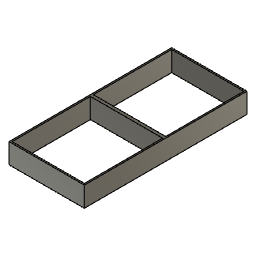
pizarra (Autodesk Fusion 360 archive; units mm, degrees)
design "Grilla F"
Autodesk Fusion 360 part; units mm, degrees
(part 1 of 4)
sketch "Sketch1" plane through (0, 0, 0) normal (0, 0, 1) x (1, 0, 0)
  line L0 (36.035, 39) -> (-36.035, 39)
  line L1 (-36.035, 39) -> (-36.035, -39)
  line L2 (-36.035, -39) -> (36.035, -39)
  line L3 (36.035, -39) -> (36.035, 39)
  line L4 (36.035, 39) -> (-36.035, -39) construction
  line L5 (-36.035, 39) -> (36.035, -39) construction
  line L6 (36.035, -39) -> (-36.035, -39)
  line L7 (-36.035, -42) -> (36.035, -42)
  line L8 (-36.035, -42) -> (36.035, -42)
  line L9 (36.035, -42) -> (36.035, -120)
  line L10 (36.035, -120) -> (-36.035, -120)
  line L11 (-36.035, -120) -> (-36.035, -42)
  line L12 (36.035, -120) -> (-36.035, -120)
  line L13 (-36.035, -121.5) -> (37.465, -121.5)
  line L14 (36.035, 39) -> (-36.035, 39)
  line L15 (-36.035, 40.5) -> (37.465, 40.5)
  line L16 (-36.035, 40.5) -> (-37.535, 40.5)
  line L17 (-37.535, 40.5) -> (-37.535, -121.5)
  line L18 (-37.535, -121.5) -> (-36.035, -121.5)
  line L19 (36.035, -120) -> (36.035, -42)
  line L20 (36.035, -39) -> (36.035, 39)
  line L21 (-36.035, -120) -> (-36.035, -42)
  line L22 (-36.035, -39) -> (-36.035, 39)
  line L23 (-37.535, -126.0665) -> (37.465, -126.0665)
  line L24 (37.465, 40.5) -> (37.465, -121.5)
  line L25 (35.965, -120) -> (35.965, -42)
  line L26 (35.965, -39) -> (35.965, 39)
  dimension "d9" = 72.07
  dimension "d10" = 78
  dimension "d11" = 3
  dimension "d12" = 78
  dimension "d14" = 159
  dimension "d17" = 1.5
  dimension "d20" = 75
  constraint horizontal L0
  constraint perpendicular L0 L1
  constraint parallel L0 L2
  constraint parallel L1 L3
  constraint coincident L4 origin
  constraint coincident L5 origin
  constraint horizontal L6
  constraint horizontal L7
  constraint horizontal L8
  constraint vertical L9
  constraint horizontal L10
  constraint vertical L11
  constraint vertical L19
  constraint horizontal L12
  constraint horizontal L13
  constraint horizontal L14
  constraint horizontal L15
  constraint horizontal L16
  constraint vertical L17
  constraint horizontal L18
  constraint vertical L21
  constraint collinear L19 L20
  constraint collinear L21 L22
  constraint perpendicular L17 L23
  constraint vertical L25
  constraint vertical L24
  constraint coincident L0 L26.end
  constraint coincident L7 L25.end
  constraint coincident L2 L26.start
  constraint collinear L25 L26
  constraint coincident L10 L25.start
  measures "d9" distance of L1.end L2.end
  measures "d10" distance of L0.end L1.end
  measures "d11" distance of L2.end L7.end
  measures "d12" distance of L7.start L10.end
  measures "d14" distance of L0.start L9.end
  measures "d17" distance of L15.start L16.end
  measures "d20" distance of L23.start L23.end
extrude "Extrude2" add sketch "Sketch1" along normal blind 20

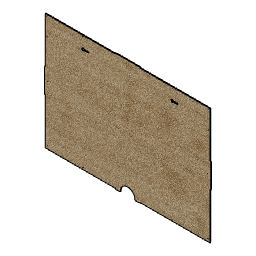
design "F.Panel Trasero.v2"
Autodesk Fusion 360 part; units mm, degrees
ref_plane "WorkPlane1" through (0, 80, 0) normal (0, 1, 0) x (0, 0, 1)
sketch "Sketch1" plane through (0, 80, 0) normal (0, 1, 0) x (1, 0, 0)
  line L0 (337.5, -238.5) -> (-337.5, 238.5) construction
  line L1 (-337.5, -238.5) -> (337.5, 238.5) construction
  line L2 (0, 0) -> (50, 0)
  line L3 (0, 0) -> (-50, 0)
  line L4 (0, 0) -> (0, -50)
  line L5 (0, 0) -> (0, 50)
  line L6 (50, -238.5) -> (50, -241.5)
  line L7 (50, -241.5) -> (-50, -241.5)
  line L8 (-50, -241.5) -> (-50, -238.5)
  line L9 (-337.5, -50) -> (-340.5, -50)
  line L10 (-340.5, -50) -> (-340.5, 50)
  line L11 (-340.5, 50) -> (-337.5, 50)
  line L12 (337.5, -50) -> (340.5, -50)
  line L13 (340.5, -50) -> (340.5, 50)
  line L14 (340.5, 50) -> (337.5, 50)
  line L15 (50, 238.5) -> (50, 241.5)
  line L16 (-50, 241.5) -> (-50, 238.5)
  arc A0 (-29.8496, 241.5) -> (29.8496, 241.5) centre (0, 238.5) ccw
  line L17 (50, 241.5) -> (29.8496, 241.5)
  line L18 (-29.8496, 241.5) -> (-50, 241.5)
  line L19 (-337.5, 238.5) -> (-50, 238.5)
  line L20 (50, 238.5) -> (337.5, 238.5)
  line L21 (337.5, 238.5) -> (337.5, 50)
  line L22 (337.5, -50) -> (337.5, -238.5)
  line L23 (337.5, -238.5) -> (50, -238.5)
  line L24 (-50, -238.5) -> (-337.5, -238.5)
  line L25 (-337.5, -238.5) -> (-337.5, -50)
  line L26 (-337.5, 50) -> (-337.5, 238.5)
  dimension "d14" = 675
  dimension "d15" = 477
  dimension "d16" = 50
  dimension "d17" = 50
  dimension "d18" = 50
  dimension "d19" = 50
  dimension "d20" = 3
  dimension "d21" = 3
  dimension "d22" = 100
  dimension "d23" = 3
  dimension "d24" = 3
  dimension "d25" = 60
  constraint horizontal L23
  constraint perpendicular L23 L25
  constraint parallel L19 L23
  constraint parallel L21 L25
  constraint coincident L0 L2.start
  constraint coincident L1 L2.start
  constraint coincident L2.start L3.start
  constraint horizontal L2
  constraint parallel L2 L3
  constraint perpendicular L3 L4
  constraint perpendicular L3 L5
  constraint vertical L6
  constraint horizontal L7
  constraint vertical L8
  constraint coincident L8.end L23
  constraint horizontal L9
  constraint vertical L10
  constraint horizontal L11
  constraint horizontal L12
  constraint vertical L13
  constraint horizontal L14
  constraint coincident L12.start L21
  constraint vertical L15
  constraint horizontal L17
  constraint vertical L16
  constraint coincident A0.start L17
  constraint collinear L17 L18
  constraint collinear L19 L20
  constraint collinear L21 L22
  constraint collinear L23 L24
  constraint collinear L25 L26
  measures "d14" distance of L0.end L1.end
  measures "d15" distance of L1.start L0.end
  measures "d16" distance of L2.start L2.end
  measures "d17" distance of L2.start L3.end
  measures "d18" distance of L2.start L4.end
  measures "d19" distance of L2.start L5.end
  measures "d20" distance of L8.end L7.end
  measures "d21" distance of L9.start L9.end
  measures "d22" distance of L9.start L11.end
  measures "d23" distance of L12.start L12.end
  measures "d24" distance of L16.end L16.start
  measures "d25" diameter of A0
extrude "Extrude3" add sketch "Sketch1" along normal blind 3
ref_plane "WorkPlane2" through (0, 80, 0) normal (0, -1, 0) x (-1, 0, 0)
sketch "Sketch2" plane through (0, 80, 0) normal (0, -1, 0) x (1, 0, 0)
  line L0 (340.5, 50) -> (337.5, 50)
  line L1 (337.5, 50) -> (337.5, 238.5)
  line L2 (337.5, 238.5) -> (50, 238.5)
  line L3 (50, 238.5) -> (50, 241.5)
  line L4 (50, 241.5) -> (-50, 241.5)
  line L5 (-50, 241.5) -> (-50, 238.5)
  line L6 (-50, 238.5) -> (-337.5, 238.5)
  line L7 (-337.5, 238.5) -> (-337.5, 50)
  line L8 (-337.5, 50) -> (-340.5, 50)
  line L9 (-340.5, 50) -> (-340.5, -50)
  line L10 (-340.5, -50) -> (-337.5, -50)
  line L11 (-337.5, -50) -> (-337.5, -238.5)
  line L12 (-337.5, -238.5) -> (-50, -238.5)
  line L13 (-50, -238.5) -> (-50, -241.5)
  line L14 (-50, -241.5) -> (-29.8496, -241.5)
  arc A0 (29.8496, -241.5) -> (-29.8496, -241.5) centre (0, -238.5) ccw
  line L15 (29.8496, -241.5) -> (50, -241.5)
  line L16 (50, -241.5) -> (50, -238.5)
  line L17 (50, -238.5) -> (337.5, -238.5)
  line L18 (337.5, -238.5) -> (337.5, -50)
  line L19 (337.5, -50) -> (340.5, -50)
  line L20 (340.5, -50) -> (340.5, 50)
ref_plane "WorkPlane3" through (0, 80, 0) normal (0, -1, 0) x (-1, 0, 0)
sketch "Sketch3" plane through (0, 80, 0) normal (0, -1, 0) x (1, 0, 0)
  circle A0 centre (-182.9674, -231.5) radius 1
  circle A1 centre (183.0674, -231.5) radius 1
  circle A2 centre (-328.5, -226.5) radius 1
  line L0 (473.5457, 191.5) -> (473.5457, 128.3996) construction
  circle A3 centre (326.5, 2.556) radius 1
  circle A4 centre (328.5, -226.5) radius 1
  line L1 (-50, 238.5) -> (-50, 241.5)
  line L2 (-340.5, -50) -> (-337.5, -50)
  line L3 (-330.5, 141.5) -> (-330.5, 159.5)
  line L4 (-330.5, 159.5) -> (-340.5, 159.5)
  line L5 (-340.5, 141.5) -> (-330.5, 141.5)
  circle A5 centre (-330.5, 232.5) radius 1
  line L6 (-330.5, 232.5) -> (-340.5, 232.5)
  line L7 (-50, 241.5) -> (-50, 238.5)
  circle A6 centre (183.022, 233.5) radius 1
  circle A7 centre (330.5, 159.5) radius 1
  circle A8 centre (330.5, 232.5) radius 1
  line L8 (330.5, 159.5) -> (338.4264, 160.0934)
  circle A9 centre (-183.0217, 233.5) radius 1
  line L9 (-330.5, 241.5) -> (-330.5, 232.5)
  line L10 (-340.5, 159.5) -> (-340.5, 141.5)
  line L11 (340.5, -50) -> (337.5, -50)
  line L12 (-337.5, -50) -> (-340.5, -50)
  line L13 (337.5, -50) -> (340.5, -50)
  line L14 (-340.5, 232.5) -> (-340.5, 241.5)
  line L15 (-340.5, 241.5) -> (-330.5, 241.5)
  circle A10 centre (-330.5, 159.3463) radius 1
  line L16 (-161.02, 186.5) -> (-178.0217, 186.5)
  line L17 (-178.0217, 190.5) -> (-161.02, 190.5)
  arc A11 (-161.02, 186.5) -> (-161.02, 190.5) centre (-161.02, 188.5) ccw
  arc A12 (-178.5672, 190.7709) -> (-178.5672, 186.2291) centre (-183.0217, 188.5) ccw
  arc A13 (205.0238, 186.5) -> (205.0238, 190.5) centre (205.0238, 188.5) ccw
  line L18 (188.022, 190.5) -> (205.0238, 190.5)
  line L19 (205.0238, 186.5) -> (188.022, 186.5)
  arc A14 (187.4765, 190.7709) -> (187.4765, 186.2291) centre (183.022, 188.5) ccw
  arc A15 (187.942, 186.5016) -> (187.4765, 186.2291) centre (187.922, 186.002) ccw
  arc A16 (187.942, 186.5016) -> (188.022, 186.5) centre (188.022, 188.5) ccw
  arc A17 (187.4765, 190.7709) -> (187.942, 190.4984) centre (187.922, 190.998) ccw
  arc A18 (188.022, 190.5) -> (187.942, 190.4984) centre (188.022, 188.5) ccw
  line L20 (-178.5672, 190.7709) -> (-178.0217, 190.5)
  line L21 (-178.5672, 186.2291) -> (-178.0217, 186.5)
  line L22 (340.5, 50) -> (337.5, 50)
  line L23 (337.5, 50) -> (337.5, 238.5)
  line L24 (337.5, 238.5) -> (50, 238.5)
  line L25 (50, 238.5) -> (50, 241.5)
  line L26 (50, 241.5) -> (-50, 241.5)
  line L27 (-50, 241.5) -> (-50, 238.5)
  line L28 (-50, 238.5) -> (-337.5, 238.5)
  line L29 (-337.5, 238.5) -> (-337.5, 50)
  line L30 (-337.5, 50) -> (-340.5, 50)
  line L31 (-340.5, 50) -> (-340.5, -50)
  line L32 (-340.5, -50) -> (-337.5, -50)
  line L33 (-337.5, -50) -> (-337.5, -238.5)
  line L34 (-337.5, -238.5) -> (-50, -238.5)
  line L35 (-50, -238.5) -> (-50, -241.5)
  line L36 (-50, -241.5) -> (-29.8496, -241.5)
  arc A19 (29.8496, -241.5) -> (-29.8496, -241.5) centre (0, -238.5) ccw
  line L37 (29.8496, -241.5) -> (50, -241.5)
  line L38 (50, -241.5) -> (50, -238.5)
  line L39 (50, -238.5) -> (337.5, -238.5)
  line L40 (337.5, -238.5) -> (337.5, -50)
  line L41 (337.5, -50) -> (340.5, -50)
  line L42 (340.5, -50) -> (340.5, 50)
  line L43 (-340.5, 241.5) -> (340.5, 241.5)
  line L44 (340.5, 241.5) -> (340.5, 141.5)
  line L45 (340.5, 141.5) -> (-340.5, 141.5)
  line L46 (-340.5, 141.5) -> (-340.5, 241.5)
  line L47 (-183.0217, 188.5) -> (-183.0217, 241.5)
  line L48 (183.022, 188.5) -> (183.022, 241.5)
  line L49 (-340.5, 3.0863) -> (-326.5, 3.0863)
  circle A20 centre (-326.5, 3.0863) radius 1
  line L50 (-337.5, -238.5) -> (-337.5, -241.5)
  line L51 (-337.5, -238.5) -> (-340.5, -238.5)
  line L52 (-337.5, -241.5) -> (-316, -241.5)
  line L53 (-340.5, -238.5) -> (-340.5, -223)
  point P0 (-3, -3)
  point P1 (-3, -3)
  point P2 (-3, -3)
  dimension "d49" = 2
  dimension "d50" = 2
  dimension "d67" = 2
  dimension "d109" = 2
  dimension "d112" = 2
  dimension "d6" = 10
  dimension "d7" = 9
  dimension "d8" = 10
  dimension "d9" = 18
  dimension "d137" = 2
  dimension "d138" = 2
  dimension "d139" = 2
  dimension "d140" = 2
  dimension "d141" = 2
  dimension "d142" = 2
  dimension "d143" = 5
  dimension "d144" = 5
  dimension "d152" = 681
  dimension "d153" = 100
  dimension "d154" = 10
  dimension "d155" = 9
  dimension "d156" = 8
  dimension "d157" = 10
  dimension "d158" = 18
  dimension "d159" = 53
  dimension "d160" = 157.4783
  dimension "d161" = 8
  dimension "d162" = 157.478
  dimension "d163" = 53
  dimension "d165" = 14
  dimension "d166" = 9
  dimension "d167" = 12
  dimension "d168" = 7
  dimension "d169" = 7
  dimension "d170" = 9
  dimension "d171" = 12
  dimension "d172" = 14
  dimension "d173" = 2
  dimension "d179" = 3
  dimension "d180" = 3
  constraint horizontal L43
  constraint vertical L44
  constraint horizontal L45
  constraint vertical L46
  constraint coincident A12.centre L47.start
  constraint coincident L43 L47.end
  constraint perpendicular L43 L47
  constraint coincident A14.centre L48.start
  constraint coincident L43 L48.end
  constraint perpendicular L43 L48
  constraint coincident L31 L49.start
  constraint perpendicular L31 L49
  constraint coincident L49.end A20.centre
  constraint coincident L33.end L34.start
  constraint perpendicular L34 L50
  constraint perpendicular L33 L51
  constraint perpendicular L50 L52
  constraint perpendicular L51 L53
  measures "d49" diameter of A0
  measures "d50" diameter of A1
  measures "d67" diameter of A2
  measures "d109" diameter of A3
  measures "d112" diameter of A4
  measures "d6" distance of L14.end L9.start
  measures "d7" distance of L6.end L14.end
  measures "d8" distance of L3.start L5.start
  measures "d9" distance of L4.end L5.start
  measures "d137" diameter of A6
  measures "d138" diameter of A9
  measures "d139" diameter of A5
  measures "d140" diameter of A10
  measures "d141" diameter of A8
  measures "d142" diameter of A7
  measures "d143" radius of A12
  measures "d144" radius of A14
  measures "d152" distance of L14.end L43.end
  measures "d153" distance of L14.end L5.start
  measures "d154" distance of A8.centre L44
  measures "d155" distance of A8.centre L43
  measures "d156" distance of A6.centre L43
  measures "d157" distance of A7.centre L44
  measures "d158" distance of A7.centre L45
  measures "d159" distance of A12.centre L43
  measures "d160" distance of A12.centre L46
  measures "d161" distance of A9.centre L43
  measures "d162" distance of A14.centre L44
  measures "d163" distance of A14.centre L43
  measures "d165" distance of A3.centre L42
  measures "d166" distance of A2.centre L33
  measures "d167" distance of A2.centre L34
  measures "d168" distance of A0.centre L34
  measures "d169" distance of A1.centre L39
  measures "d170" distance of A4.centre L40
  measures "d171" distance of A4.centre L39
  measures "d172" distance of L49.start L49.end
  measures "d173" diameter of A20
  measures "d179" distance of L33.end L50.end
  measures "d180" distance of L33.end L51.end
extrude "Extrude4" cut sketch "Sketch3" against normal blind 50 contours A0 | A1 | A2 | A3 | A4 | A5 L6 L9 | A5 L6 L9 | L3 L4 A10 | L3 L4 A10 | A6 L48 | A6 L48 | A7 | A8 | A9 L47 | A9 L47 | L16 L17 A11 A12 L20 L21 | A13 L18 L19 A14 A15 A16 A17 A18 | A20
ref_plane "WorkPlane4" through (0, 80, 0) normal (0, -1, 0) x (-1, 0, 0)
sketch "Sketch5" plane through (0, 80, 0) normal (0, -1, 0) x (1, 0, 0)
  circle A0 centre (330.5, 232.5) radius 1
  circle A1 centre (-330.5, 232.5) radius 1
  circle A2 centre (-328.5, -226.5) radius 1
  circle A3 centre (-182.9674, -231.5) radius 1
  circle A4 centre (-330.5, 159.3463) radius 1
  circle A5 centre (330.5, 159.5) radius 1
  line L0 (-178.0217, 186.5) -> (-178.5672, 186.2291)
  arc A6 (-178.5672, 190.7709) -> (-178.5672, 186.2291) centre (-183.0217, 188.5) ccw
  line L1 (-178.5672, 190.7709) -> (-178.0217, 190.5)
  line L2 (-178.0217, 190.5) -> (-161.02, 190.5)
  arc A7 (-161.02, 186.5) -> (-161.02, 190.5) centre (-161.02, 188.5) ccw
  line L3 (-161.02, 186.5) -> (-178.0217, 186.5)
  circle A8 centre (-183.0217, 233.5) radius 1
  circle A9 centre (326.5, 2.556) radius 1
  circle A10 centre (183.0674, -231.5) radius 1
  circle A11 centre (328.5, -226.5) radius 1
  circle A12 centre (183.022, 233.5) radius 1
  line L4 (188.022, 190.5) -> (205.0238, 190.5)
  arc A13 (205.0238, 186.5) -> (205.0238, 190.5) centre (205.0238, 188.5) ccw
  line L5 (205.0238, 186.5) -> (188.022, 186.5)
  arc A14 (187.942, 186.5016) -> (188.022, 186.5) centre (188.022, 188.5) ccw
  arc A15 (187.942, 186.5016) -> (187.4765, 186.2291) centre (187.922, 186.002) ccw
  arc A16 (187.4765, 190.7709) -> (187.4765, 186.2291) centre (183.022, 188.5) ccw
  arc A17 (187.4765, 190.7709) -> (187.942, 190.4984) centre (187.922, 190.998) ccw
  arc A18 (188.022, 190.5) -> (187.942, 190.4984) centre (188.022, 188.5) ccw
  line L6 (340.5, 50) -> (337.5, 50)
  line L7 (337.5, 50) -> (337.5, 238.5)
  line L8 (337.5, 238.5) -> (50, 238.5)
  line L9 (50, 238.5) -> (50, 241.5)
  line L10 (50, 241.5) -> (-50, 241.5)
  line L11 (-50, 241.5) -> (-50, 238.5)
  line L12 (-50, 238.5) -> (-337.5, 238.5)
  line L13 (-337.5, 238.5) -> (-337.5, 50)
  line L14 (-337.5, 50) -> (-340.5, 50)
  line L15 (-340.5, 50) -> (-340.5, -50)
  line L16 (-340.5, -50) -> (-337.5, -50)
  line L17 (-337.5, -50) -> (-337.5, -238.5)
  line L18 (-337.5, -238.5) -> (-50, -238.5)
  line L19 (-50, -238.5) -> (-50, -241.5)
  line L20 (-50, -241.5) -> (-29.8496, -241.5)
  arc A19 (29.8496, -241.5) -> (-29.8496, -241.5) centre (0, -238.5) ccw
  line L21 (29.8496, -241.5) -> (50, -241.5)
  line L22 (50, -241.5) -> (50, -238.5)
  line L23 (50, -238.5) -> (337.5, -238.5)
  line L24 (337.5, -238.5) -> (337.5, -50)
  line L25 (337.5, -50) -> (340.5, -50)
  line L26 (340.5, -50) -> (340.5, 50)
  line L27 (-337.5, 238.5) -> (-337.5, 241.5)
  line L28 (-337.5, 238.5) -> (-340.5, 238.5)
  line L29 (337.5, 238.5) -> (340.5, 238.5)
  line L30 (-340.5, 241.5) -> (340.5, 241.5)
  line L31 (340.5, 241.5) -> (340.5, 141.5)
  line L32 (340.5, 141.5) -> (-340.5, 141.5)
  line L33 (-340.5, 141.5) -> (-340.5, 241.5)
  circle A20 centre (-326.5, 3.0863) radius 1
  dimension "d174" = 3
  dimension "d175" = 3
  dimension "d176" = 3
  dimension "d177" = 100
  dimension "d178" = 681
  constraint coincident L12.end L13.start
  constraint perpendicular L12 L27
  constraint perpendicular L13 L28
  constraint coincident L7.end L8.start
  constraint perpendicular L7 L29
  constraint horizontal L30
  constraint vertical L31
  constraint horizontal L32
  constraint vertical L33
  measures "d174" distance of L12.end L27.end
  measures "d175" distance of L12.end L28.end
  measures "d176" distance of L7.end L29.end
  measures "d177" distance of L30.start L32.end
  measures "d178" distance of L30.start L30.end

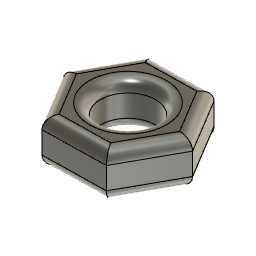
design "N.Perno Alen.v2"
Autodesk Fusion 360 part; units mm, degrees
sketch "Sketch1" plane through (0, 0, 0) normal (0, 0, 1) x (1, 0, 0)
  line L0 (-1.4906, 2.4721) -> (-2.8862, -0.0549)
  line L1 (-2.8862, -0.0549) -> (-1.3956, -2.527)
  line L2 (-1.3956, -2.527) -> (1.4906, -2.4721)
  line L3 (1.4906, -2.4721) -> (2.8862, 0.0549)
  line L4 (2.8862, 0.0549) -> (1.3956, 2.527)
  line L5 (1.3956, 2.527) -> (-1.4906, 2.4721)
  circle A0 centre (0, 0) radius 1.25
  dimension "d1" = 2.5
  dimension "d2" = 2.5
  constraint coincident A0.centre origin
  measures "d1" distance of A0.centre L5
  measures "d2" diameter of A0
extrude "Extrude1" add sketch "Sketch1" along normal blind 2
fillet "Fillet1" radius 0.5 1 faces at (0.0628, -2.0819, 2)
fillet "Fillet2" radius 0.5 1 faces at (0.0628, -2.0819, 0)

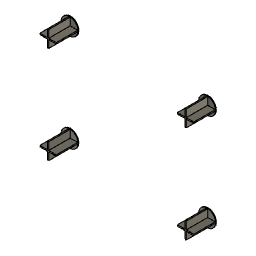
design "Cruceta para fondo.v3"
Autodesk Fusion 360 part; units mm, degrees
sketch "Sketch1" plane through (0, 0, 0) normal (0, 1, 0) x (1, 0, 0)
  line L0 (337.5, -238.5) -> (-337.5, -238.5)
  line L1 (-337.5, -238.5) -> (-337.5, 238.5)
  line L2 (-337.5, 238.5) -> (337.5, 238.5)
  line L3 (337.5, 238.5) -> (337.5, -238.5)
  line L4 (0, 0) -> (-163.3332, -115.4221) construction
  circle A0 centre (-163.3332, -115.4221) radius 20
  circle A1 centre (163.3332, -115.4221) radius 20
  circle A2 centre (-163.3332, 115.4221) radius 20
  circle A3 centre (163.3332, 115.4221) radius 20
  line L5 (-161.8332, -134.9221) -> (-164.8332, -134.9221)
  line L6 (-164.8332, -95.9221) -> (-161.8332, -95.9221)
  line L7 (-161.8332, -134.9221) -> (-164.8332, -95.9221) construction
  line L8 (-164.8332, -134.9221) -> (-161.8332, -95.9221) construction
  line L9 (-182.8332, -116.9221) -> (-182.8332, -113.9221)
  line L10 (-143.8332, -113.9221) -> (-143.8332, -116.9221)
  line L11 (-143.8332, -116.9221) -> (-182.8332, -113.9221) construction
  line L12 (-182.8332, -116.9221) -> (-143.8332, -113.9221) construction
  line L13 (-337.5, -238.5) -> (-164.8332, -116.4821) construction
  line L14 (-163.3332, -115.4221) -> (337.5, 238.5) construction
  line L15 (-164.8332, -134.9221) -> (-164.8332, -116.9221) construction
  line L16 (-143.8332, -116.9221) -> (-161.8332, -116.9221) construction
  line L17 (-164.8332, -116.9221) -> (-182.8332, -116.9221) construction
  line L18 (-161.8332, -116.9221) -> (-161.8332, -134.9221) construction
  line L19 (-161.8332, -95.9221) -> (-161.8332, -113.9221) construction
  line L20 (-182.8332, -113.9221) -> (-164.8332, -113.9221) construction
  line L21 (-161.8332, -113.9221) -> (-143.8332, -113.9221) construction
  line L22 (-164.8332, -113.9221) -> (-164.8332, -95.9221) construction
  point P0 (-163.3332, -115.4221)
  point P1 (-163.3332, -115.4221)
  dimension "d1" = 675
  dimension "d2" = 477
  dimension "d3" = 200
  dimension "d4" = 200
  dimension "d5" = 200
  dimension "d6" = 200
  dimension "d7" = 40
  dimension "d8" = 40
  dimension "d9" = 40
  dimension "d10" = 40
  dimension "d11" = 3
  dimension "d12" = 39
  dimension "d13" = 3
  dimension "d14" = 39
  constraint horizontal L0
  constraint perpendicular L0 L1
  constraint parallel L0 L2
  constraint parallel L1 L3
  constraint coincident L4.start L13
  constraint coincident L4.start origin
  constraint coincident P1 L13
  constraint coincident P1 P0
  constraint horizontal L5
  constraint perpendicular L5 L15
  constraint parallel L5 L6
  constraint parallel L15 L19
  constraint coincident L7 P1
  constraint coincident L8 P1
  constraint horizontal L16
  constraint perpendicular L9 L16
  constraint parallel L16 L20
  constraint parallel L9 L10
  constraint coincident L11 P1
  constraint coincident L12 P1
  constraint collinear L13 L14
  constraint coincident L15.end L16
  constraint collinear L16 L17
  constraint coincident L16.end L19
  constraint collinear L18 L19
  constraint coincident L19.end L20
  constraint collinear L20 L21
  measures "d1" distance of L1.end L2.end
  measures "d2" distance of L0.end L1.end
  measures "d3" distance of L4.start P1
  measures "d4" distance of L4.start A1.centre
  measures "d5" distance of L4.start A2.centre
  measures "d6" distance of L4.start A3.centre
  measures "d7" diameter of A0
  measures "d8" diameter of A1
  measures "d9" diameter of A2
  measures "d10" diameter of A3
  measures "d11" distance of L6.start L6.end
  measures "d12" distance of L9.end L10.start
  measures "d13" distance of L9.start L9.end
  measures "d14" distance of L5.start L6.end
extrude "Extrude1" add sketch "Sketch1" along normal blind 2 contours A0 | A1 | A2 | A3 makes body 1 at (-164.4526, 0, -120.9941) makes body 2 at (160.7303, 0, 116.3496) makes body 3 at (-163.5939, 0, 118.7453) makes body 4 at (162.2137, 0, -120.9941)
ref_plane "WorkPlane1" through (-163.3332, 0, 115.4221) normal (0, -1, 0) x (-1, 0, 0)
sketch "Sketch2" plane through (-163.3332, 0, 115.4221) normal (0, -1, 0) x (1, 0, 0)
  line L0 (1.5, 19.5) -> (-1.5, 19.5)
  line L1 (-1.5, 19.5) -> (-1.5, 1.5)
  line L2 (1.5, 1.5) -> (1.5, 19.5)
  line L3 (-1.5, 1.5) -> (-19.5, 1.5)
  line L4 (-19.5, 1.5) -> (-19.5, -1.5)
  line L5 (-19.5, -1.5) -> (-1.5, -1.5)
  line L6 (19.5, 1.5) -> (1.5, 1.5)
  line L7 (19.5, -1.5) -> (19.5, 1.5)
  line L8 (1.5, -1.5) -> (19.5, -1.5)
  line L9 (1.5, -19.5) -> (1.5, -1.5)
  line L10 (-1.5, -19.5) -> (1.5, -19.5)
  line L11 (-1.5, -1.5) -> (-1.5, -19.5)
  line L12 (1.5, -1.5) -> (19.5, -1.5)
  line L13 (-1.5, 1.5) -> (-19.5, 1.5)
  line L14 (1.5, 19.5) -> (-1.5, 19.5)
  line L15 (-19.5, -1.5) -> (-1.5, -1.5)
  line L16 (-1.5, -1.5) -> (-1.5, -19.5)
  line L17 (19.5, 1.5) -> (1.5, 1.5)
  line L18 (1.5, 1.5) -> (1.5, 19.5)
  line L19 (19.5, -1.5) -> (19.5, 1.5)
  line L20 (-1.5, -19.5) -> (1.5, -19.5)
  line L21 (-1.5, 19.5) -> (-1.5, 1.5)
  line L22 (1.5, -19.5) -> (1.5, -1.5)
  line L23 (-19.5, 1.5) -> (-19.5, -1.5)
  circle A0 centre (0, 0) radius 20
  circle A1 centre (326.6664, 0) radius 20
  circle A2 centre (326.6664, -230.8443) radius 20
  circle A3 centre (0, -230.8443) radius 20
  line L24 (325.1664, -19.5) -> (328.1664, -19.5)
  line L25 (325.1664, 19.5) -> (325.1664, 1.5)
  line L26 (307.1664, -1.5) -> (325.1664, -1.5)
  line L27 (307.1664, -1.5) -> (325.1664, -1.5)
  line L28 (325.1664, -1.5) -> (325.1664, -19.5)
  line L29 (346.1664, -1.5) -> (346.1664, 1.5)
  line L30 (328.1664, -19.5) -> (328.1664, -1.5)
  line L31 (307.1664, 1.5) -> (307.1664, -1.5)
  line L32 (346.1664, 1.5) -> (328.1664, 1.5)
  line L33 (328.1664, 19.5) -> (325.1664, 19.5)
  line L34 (346.1664, -1.5) -> (346.1664, 1.5)
  line L35 (328.1664, 1.5) -> (328.1664, 19.5)
  circle A4 centre (326.6664, 0) radius 20
  line L36 (346.1664, 1.5) -> (328.1664, 1.5)
  line L37 (325.1664, 1.5) -> (307.1664, 1.5)
  line L38 (325.1664, -19.5) -> (328.1664, -19.5)
  line L39 (325.1664, 19.5) -> (325.1664, 1.5)
  line L40 (328.1664, -1.5) -> (346.1664, -1.5)
  line L41 (328.1664, -19.5) -> (328.1664, -1.5)
  line L42 (328.1664, 19.5) -> (325.1664, 19.5)
  line L43 (328.1664, 1.5) -> (328.1664, 19.5)
  line L44 (325.1664, 1.5) -> (307.1664, 1.5)
  line L45 (328.1664, -1.5) -> (346.1664, -1.5)
  line L46 (307.1664, 1.5) -> (307.1664, -1.5)
  line L47 (325.1664, -1.5) -> (325.1664, -19.5)
  line L48 (328.1664, -211.3443) -> (325.1664, -211.3443)
  line L49 (346.1664, -232.3443) -> (346.1664, -229.3443)
  line L50 (328.1664, -229.3443) -> (328.1664, -211.3443)
  line L51 (325.1664, -232.3443) -> (325.1664, -250.3443)
  line L52 (307.1664, -232.3443) -> (325.1664, -232.3443)
  circle A5 centre (326.6664, -230.8443) radius 20
  line L53 (328.1664, -211.3443) -> (325.1664, -211.3443)
  line L54 (307.1664, -229.3443) -> (307.1664, -232.3443)
  line L55 (307.1664, -229.3443) -> (307.1664, -232.3443)
  line L56 (325.1664, -250.3443) -> (328.1664, -250.3443)
  line L57 (328.1664, -250.3443) -> (328.1664, -232.3443)
  line L58 (307.1664, -232.3443) -> (325.1664, -232.3443)
  line L59 (346.1664, -229.3443) -> (328.1664, -229.3443)
  line L60 (328.1664, -229.3443) -> (328.1664, -211.3443)
  line L61 (328.1664, -232.3443) -> (346.1664, -232.3443)
  line L62 (325.1664, -232.3443) -> (325.1664, -250.3443)
  line L63 (328.1664, -250.3443) -> (328.1664, -232.3443)
  line L64 (325.1664, -211.3443) -> (325.1664, -229.3443)
  line L65 (325.1664, -229.3443) -> (307.1664, -229.3443)
  line L66 (325.1664, -211.3443) -> (325.1664, -229.3443)
  line L67 (325.1664, -229.3443) -> (307.1664, -229.3443)
  line L68 (346.1664, -229.3443) -> (328.1664, -229.3443)
  circle A6 centre (326.6664, -230.8443) radius 20
  line L69 (325.1664, -250.3443) -> (328.1664, -250.3443)
  line L70 (346.1664, -232.3443) -> (346.1664, -229.3443)
  line L71 (328.1664, -232.3443) -> (346.1664, -232.3443)
  line L72 (1.5, -211.3443) -> (-1.5, -211.3443)
  line L73 (19.5, -232.3443) -> (19.5, -229.3443)
  line L74 (1.5, -229.3443) -> (1.5, -211.3443)
  line L75 (-1.5, -232.3443) -> (-1.5, -250.3443)
  line L76 (-19.5, -232.3443) -> (-1.5, -232.3443)
  circle A7 centre (0, -230.8443) radius 20
  line L77 (1.5, -211.3443) -> (-1.5, -211.3443)
  line L78 (-19.5, -229.3443) -> (-19.5, -232.3443)
  line L79 (-19.5, -229.3443) -> (-19.5, -232.3443)
  line L80 (-1.5, -250.3443) -> (1.5, -250.3443)
  line L81 (1.5, -250.3443) -> (1.5, -232.3443)
  line L82 (-19.5, -232.3443) -> (-1.5, -232.3443)
  line L83 (19.5, -229.3443) -> (1.5, -229.3443)
  line L84 (1.5, -229.3443) -> (1.5, -211.3443)
  line L85 (1.5, -232.3443) -> (19.5, -232.3443)
  line L86 (-1.5, -232.3443) -> (-1.5, -250.3443)
  line L87 (1.5, -250.3443) -> (1.5, -232.3443)
  line L88 (-1.5, -211.3443) -> (-1.5, -229.3443)
  line L89 (-1.5, -229.3443) -> (-19.5, -229.3443)
  line L90 (-1.5, -211.3443) -> (-1.5, -229.3443)
  line L91 (-1.5, -229.3443) -> (-19.5, -229.3443)
  line L92 (19.5, -229.3443) -> (1.5, -229.3443)
  circle A8 centre (0, -230.8443) radius 20
  line L93 (-1.5, -250.3443) -> (1.5, -250.3443)
  line L94 (19.5, -232.3443) -> (19.5, -229.3443)
  line L95 (1.5, -232.3443) -> (19.5, -232.3443)
  point P0 (306.6664, -230.8443)
  point P1 (326.6664, 0)
  point P2 (326.6664, 0)
  point P3 (326.6664, -230.8443)
  point P4 (326.6664, -230.8443)
  point P5 (0, -230.8443)
  point P6 (0, -230.8443)
extrude "Extrude2" add sketch "Sketch2" along normal blind 51 contours L0 L1 L2 L3 L4 L5 L6 L7 L8 L9 L10 L11 L12 L13 L14 L15 L16 L17 L18 L19 L20 L21 L22 L23 | L24 L25 L26 L27 L28 L29 L30 L31 L32 L33 L34 L35 L36 L37 L38 L39 L40 L41 L42 L43 L44 L45 L46 L47 | L48 L49 L50 L51 L52 L53 L54 L55 L56 L57 L58 L59 L60 L61 L62 L63 L64 L65 L66 L67 L68 L69 L70 L71 bodies 2 3 4
extrude "Extrude3" add sketch "Sketch2" along normal blind 51 contours L72 L73 L74 L75 L76 L77 L78 L79 L80 L81 L82 L83 L84 L85 L86 L87 L88 L89 L90 L91 L92 L93 L94 L95 bodies 1

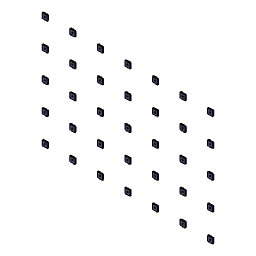
design "onjunto piezas perno"
Autodesk Fusion 360 part; units mm, degrees
sketch "Sketch1" plane through (0, 0, 0) normal (0, 1, 0) x (1, 0, 0)
  circle A0 centre (252, -728) radius 1.75
  circle A1 centre (252, -647) radius 1.75
  line L0 (325.5, -735.5) -> (340.5, -735.5)
  circle A2 centre (252, -566) radius 1.75
  line L1 (259.5, -654.5) -> (259.5, -639.5)
  line L2 (340.5, -636.5) -> (340.5, -639.5)
  line L3 (340.5, -639.5) -> (325.5, -639.5)
  line L4 (340.5, -720.5) -> (325.5, -720.5)
  line L5 (97.5, -735.5) -> (97.5, -720.5)
  circle A3 centre (252, -809) radius 1.75
  line L6 (-340.5, -636.5) -> (340.5, -636.5) construction
  line L7 (178.5, -735.5) -> (178.5, -720.5)
  line L8 (-340.5, -882.5) -> (340.5, -882.5) construction
  line L9 (325.5, -816.5) -> (340.5, -816.5)
  line L10 (-340.5, -960.5) -> (340.5, -960.5) construction
  line L11 (-340.5, -801.5) -> (340.5, -801.5) construction
  line L12 (262.5, -963.5) -> (262.5, -1041.5) construction
  line L13 (340.5, -801.5) -> (340.5, -879.5)
  circle A4 centre (171, -566) radius 1.75
  line L14 (325.5, -801.5) -> (325.5, -816.5)
  line L15 (244.5, -816.5) -> (259.5, -816.5)
  line L16 (340.5, -816.5) -> (340.5, -801.5)
  line L17 (340.5, -717.5) -> (-340.5, -717.5) construction
  line L18 (-340.5, -639.5) -> (340.5, -639.5) construction
  line L19 (19.5, -1041.5) -> (97.5, -1041.5) construction
  line L20 (340.5, -882.5) -> (-340.5, -882.5) construction
  line L21 (-340.5, -558.5) -> (340.5, -558.5) construction
  circle A5 centre (252, -890) radius 1.75
  line L22 (259.5, -897.5) -> (259.5, -882.5)
  line L23 (340.5, -1041.5) -> (-340.5, -1041.5) construction
  line L24 (-340.5, -798.5) -> (340.5, -798.5) construction
  line L25 (100.5, -558.5) -> (97.5, -558.5)
  line L26 (340.5, -798.5) -> (-340.5, -798.5) construction
  line L27 (-340.5, -720.5) -> (340.5, -720.5) construction
  line L28 (16.5, -720.5) -> (1.5, -720.5)
  line L29 (-226.5, -1041.5) -> (-223.5, -1041.5) construction
  line L30 (82.5, -816.5) -> (97.5, -816.5)
  circle A6 centre (171, -890) radius 1.75
  line L31 (-340.5, -639.5) -> (-340.5, -636.5)
  line L32 (97.5, -1041.5) -> (100.5, -1041.5) construction
  line L33 (-340.5, -882.5) -> (-340.5, -879.5)
  circle A7 centre (-153, -809) radius 1.75
  circle A8 centre (-72, -728) radius 1.75
  line L34 (16.5, -816.5) -> (16.5, -801.5)
  line L35 (-64.5, -1041.5) -> (-64.5, -963.5) construction
  line L36 (-160.5, -720.5) -> (-160.5, -735.5)
  line L37 (-160.5, -816.5) -> (-145.5, -816.5)
  circle A9 centre (-72, -890) radius 1.75
  line L38 (1.5, -882.5) -> (1.5, -897.5)
  line L39 (-223.5, -1041.5) -> (-145.5, -1041.5) construction
  line L40 (-145.5, -897.5) -> (-145.5, -882.5)
  line L41 (178.5, -1041.5) -> (181.5, -1041.5) construction
  line L42 (-64.5, -558.5) -> (-79.5, -558.5)
  line L43 (178.5, -1041.5) -> (178.5, -963.5) construction
  line L44 (-145.5, -573.5) -> (-145.5, -558.5)
  line L45 (-145.5, -963.5) -> (-223.5, -963.5)
  circle A10 centre (-153, -566) radius 1.75
  line L46 (178.5, -816.5) -> (178.5, -801.5)
  line L47 (-64.5, -573.5) -> (-64.5, -558.5)
  line L48 (-160.5, -801.5) -> (-160.5, -816.5)
  line L49 (-340.5, -1041.5) -> (-226.5, -1041.5) construction
  line L50 (-145.5, -558.5) -> (-160.5, -558.5)
  line L51 (-160.5, -558.5) -> (-160.5, -573.5)
  line L52 (-61.5, -963.5) -> (-61.5, -1041.5) construction
  line L53 (-142.5, -558.5) -> (-145.5, -558.5)
  line L54 (-160.5, -654.5) -> (-145.5, -654.5)
  line L55 (163.5, -897.5) -> (178.5, -897.5)
  circle A11 centre (-72, -566) radius 1.75
  circle A12 centre (-153, -728) radius 1.75
  line L56 (-145.5, -882.5) -> (-160.5, -882.5)
  line L57 (-340.5, -801.5) -> (-340.5, -798.5)
  line L58 (-145.5, -1041.5) -> (-142.5, -1041.5) construction
  line L59 (-79.5, -573.5) -> (-64.5, -573.5)
  line L60 (82.5, -882.5) -> (82.5, -897.5)
  line L61 (181.5, -963.5) -> (181.5, -1041.5) construction
  line L62 (-160.5, -573.5) -> (-145.5, -573.5)
  line L63 (-145.5, -720.5) -> (-160.5, -720.5)
  line L64 (16.5, -654.5) -> (16.5, -639.5)
  line L65 (16.5, -882.5) -> (1.5, -882.5)
  circle A13 centre (9, -890) radius 1.75
  line L66 (-160.5, -882.5) -> (-160.5, -897.5)
  line L67 (16.5, -963.5) -> (-61.5, -963.5)
  line L68 (100.5, -963.5) -> (100.5, -1041.5) construction
  line L69 (-64.5, -654.5) -> (-64.5, -639.5)
  circle A14 centre (9, -728) radius 1.75
  line L70 (16.5, -639.5) -> (1.5, -639.5)
  line L71 (16.5, -735.5) -> (16.5, -720.5)
  line L72 (-64.5, -639.5) -> (-79.5, -639.5)
  circle A15 centre (-72, -809) radius 1.75
  line L73 (-61.5, -1041.5) -> (16.5, -1041.5) construction
  line L74 (1.5, -558.5) -> (1.5, -573.5)
  line L75 (-340.5, -879.5) -> (-340.5, -801.5)
  line L76 (-64.5, -1041.5) -> (-61.5, -1041.5) construction
  line L77 (1.5, -816.5) -> (16.5, -816.5)
  line L78 (-64.5, -897.5) -> (-64.5, -882.5)
  line L79 (16.5, -1041.5) -> (19.5, -1041.5) construction
  line L80 (-79.5, -735.5) -> (-64.5, -735.5)
  line L81 (1.5, -897.5) -> (16.5, -897.5)
  line L82 (-64.5, -882.5) -> (-79.5, -882.5)
  line L83 (16.5, -1041.5) -> (16.5, -963.5) construction
  line L84 (-160.5, -897.5) -> (-145.5, -897.5)
  circle A16 centre (9, -566) radius 1.75
  line L85 (-145.5, -816.5) -> (-145.5, -801.5)
  line L86 (-145.5, -1041.5) -> (-145.5, -963.5) construction
  line L87 (-79.5, -897.5) -> (-64.5, -897.5)
  line L88 (-142.5, -963.5) -> (-142.5, -1041.5) construction
  line L89 (-79.5, -720.5) -> (-79.5, -735.5)
  circle A17 centre (9, -809) radius 1.75
  line L90 (-79.5, -882.5) -> (-79.5, -897.5)
  line L91 (-61.5, -558.5) -> (-64.5, -558.5)
  circle A18 centre (-72, -647) radius 1.75
  line L92 (1.5, -801.5) -> (1.5, -816.5)
  line L93 (-340.5, -960.5) -> (-340.5, -882.5)
  line L94 (-79.5, -816.5) -> (-64.5, -816.5)
  line L95 (-340.5, -963.5) -> (-340.5, -960.5)
  line L96 (-64.5, -816.5) -> (-64.5, -801.5)
  circle A19 centre (-153, -890) radius 1.75
  line L97 (16.5, -558.5) -> (1.5, -558.5)
  line L98 (1.5, -639.5) -> (1.5, -654.5)
  line L99 (16.5, -897.5) -> (16.5, -882.5)
  line L100 (-145.5, -801.5) -> (-160.5, -801.5)
  line L101 (19.5, -558.5) -> (16.5, -558.5)
  line L102 (-223.5, -963.5) -> (-223.5, -1041.5) construction
  line L103 (-79.5, -654.5) -> (-64.5, -654.5)
  line L104 (244.5, -654.5) -> (259.5, -654.5)
  line L105 (340.5, -654.5) -> (340.5, -639.5)
  line L106 (259.5, -720.5) -> (244.5, -720.5)
  line L107 (259.5, -735.5) -> (259.5, -720.5)
  line L108 (259.5, -573.5) -> (259.5, -558.5)
  line L109 (244.5, -573.5) -> (259.5, -573.5)
  line L110 (325.5, -558.5) -> (325.5, -573.5)
  line L111 (340.5, -717.5) -> (340.5, -720.5)
  line L112 (259.5, -558.5) -> (244.5, -558.5)
  line L113 (325.5, -639.5) -> (325.5, -654.5)
  line L114 (340.5, -558.5) -> (325.5, -558.5)
  line L115 (340.5, -639.5) -> (340.5, -717.5)
  line L116 (325.5, -654.5) -> (340.5, -654.5)
  line L117 (340.5, -639.5) -> (-340.5, -639.5) construction
  line L118 (97.5, -573.5) -> (97.5, -558.5)
  line L119 (163.5, -573.5) -> (178.5, -573.5)
  line L120 (82.5, -573.5) -> (97.5, -573.5)
  line L121 (82.5, -639.5) -> (82.5, -654.5)
  circle A20 centre (171, -728) radius 1.75
  line L122 (163.5, -735.5) -> (178.5, -735.5)
  circle A21 centre (171, -647) radius 1.75
  line L123 (82.5, -720.5) -> (82.5, -735.5)
  line L124 (178.5, -654.5) -> (178.5, -639.5)
  line L125 (178.5, -639.5) -> (163.5, -639.5)
  line L126 (97.5, -720.5) -> (82.5, -720.5)
  line L127 (340.5, -720.5) -> (-340.5, -720.5) construction
  line L128 (97.5, -558.5) -> (82.5, -558.5)
  line L129 (163.5, -558.5) -> (163.5, -573.5)
  line L130 (181.5, -558.5) -> (178.5, -558.5)
  line L131 (178.5, -558.5) -> (163.5, -558.5)
  line L132 (82.5, -735.5) -> (97.5, -735.5)
  line L133 (82.5, -558.5) -> (82.5, -573.5)
  line L134 (178.5, -573.5) -> (178.5, -558.5)
  line L135 (163.5, -639.5) -> (163.5, -654.5)
  line L136 (97.5, -654.5) -> (97.5, -639.5)
  line L137 (178.5, -720.5) -> (163.5, -720.5)
  line L138 (163.5, -654.5) -> (178.5, -654.5)
  line L139 (163.5, -720.5) -> (163.5, -735.5)
  circle A22 centre (90, -566) radius 1.75
  line L140 (325.5, -573.5) -> (340.5, -573.5)
  line L141 (244.5, -735.5) -> (259.5, -735.5)
  circle A23 centre (333, -566) radius 1.75
  line L142 (262.5, -558.5) -> (259.5, -558.5)
  line L143 (259.5, -639.5) -> (244.5, -639.5)
  circle A24 centre (333, -647) radius 1.75
  circle A25 centre (333, -728) radius 1.75
  line L144 (340.5, -573.5) -> (340.5, -558.5)
  line L145 (244.5, -639.5) -> (244.5, -654.5)
  line L146 (340.5, -735.5) -> (340.5, -720.5)
  line L147 (244.5, -558.5) -> (244.5, -573.5)
  line L148 (244.5, -720.5) -> (244.5, -735.5)
  line L149 (97.5, -639.5) -> (82.5, -639.5)
  line L150 (325.5, -720.5) -> (325.5, -735.5)
  circle A26 centre (90, -728) radius 1.75
  circle A27 centre (90, -647) radius 1.75
  line L151 (82.5, -654.5) -> (97.5, -654.5)
  line L152 (-226.5, -1041.5) -> (-226.5, -558.5) construction
  line L153 (100.5, -1041.5) -> (178.5, -1041.5) construction
  line L154 (244.5, -882.5) -> (244.5, -897.5)
  line L155 (244.5, -801.5) -> (244.5, -816.5)
  line L156 (340.5, -882.5) -> (325.5, -882.5)
  line L157 (-340.5, -1041.5) -> (-340.5, -558.5) construction
  line L158 (-340.5, -798.5) -> (-340.5, -720.5)
  line L159 (-340.5, -879.5) -> (340.5, -879.5) construction
  line L160 (259.5, -882.5) -> (244.5, -882.5)
  line L161 (340.5, -879.5) -> (-340.5, -879.5) construction
  line L162 (340.5, -720.5) -> (340.5, -798.5)
  line L163 (340.5, -801.5) -> (-340.5, -801.5) construction
  line L164 (100.5, -1041.5) -> (100.5, -558.5) construction
  line L165 (244.5, -897.5) -> (259.5, -897.5)
  line L166 (97.5, -963.5) -> (19.5, -963.5)
  line L167 (259.5, -558.5) -> (259.5, -1041.5) construction
  line L168 (-142.5, -1041.5) -> (-142.5, -558.5) construction
  line L169 (340.5, -960.5) -> (340.5, -963.5)
  line L170 (-340.5, -558.5) -> (-340.5, -1041.5) construction
  line L171 (97.5, -558.5) -> (97.5, -1041.5) construction
  line L172 (340.5, -879.5) -> (340.5, -882.5)
  line L173 (259.5, -963.5) -> (181.5, -963.5)
  line L174 (-223.5, -1041.5) -> (-223.5, -558.5) construction
  line L175 (181.5, -1041.5) -> (181.5, -558.5) construction
  line L176 (181.5, -1041.5) -> (259.5, -1041.5) construction
  line L177 (340.5, -960.5) -> (-340.5, -960.5) construction
  line L178 (16.5, -558.5) -> (16.5, -1041.5) construction
  line L179 (-226.5, -558.5) -> (-226.5, -1041.5) construction
  line L180 (340.5, -882.5) -> (340.5, -960.5)
  line L181 (-145.5, -558.5) -> (-145.5, -1041.5) construction
  line L182 (163.5, -816.5) -> (178.5, -816.5)
  line L183 (325.5, -897.5) -> (340.5, -897.5)
  line L184 (178.5, -558.5) -> (178.5, -1041.5) construction
  line L185 (340.5, -558.5) -> (340.5, -1041.5) construction
  line L186 (-61.5, -1041.5) -> (-61.5, -558.5) construction
  line L187 (-64.5, -558.5) -> (-64.5, -1041.5) construction
  line L188 (-340.5, -717.5) -> (340.5, -717.5) construction
  line L189 (340.5, -963.5) -> (-340.5, -963.5) construction
  line L190 (97.5, -882.5) -> (82.5, -882.5)
  line L191 (340.5, -897.5) -> (340.5, -882.5)
  line L192 (262.5, -1041.5) -> (262.5, -558.5) construction
  line L193 (340.5, -798.5) -> (340.5, -801.5)
  line L194 (259.5, -816.5) -> (259.5, -801.5)
  line L195 (259.5, -1041.5) -> (262.5, -1041.5) construction
  line L196 (178.5, -882.5) -> (163.5, -882.5)
  line L197 (82.5, -897.5) -> (97.5, -897.5)
  line L198 (19.5, -1041.5) -> (19.5, -558.5) construction
  line L199 (178.5, -801.5) -> (163.5, -801.5)
  line L200 (340.5, -963.5) -> (262.5, -963.5)
  line L201 (-340.5, -720.5) -> (-340.5, -717.5)
  line L202 (-64.5, -720.5) -> (-79.5, -720.5)
  line L203 (178.5, -897.5) -> (178.5, -882.5)
  line L204 (-64.5, -963.5) -> (-142.5, -963.5)
  line L205 (1.5, -573.5) -> (16.5, -573.5)
  line L206 (97.5, -1041.5) -> (97.5, -963.5) construction
  line L207 (178.5, -963.5) -> (100.5, -963.5)
  line L208 (325.5, -882.5) -> (325.5, -897.5)
  line L209 (-145.5, -639.5) -> (-160.5, -639.5)
  circle A28 centre (90, -890) radius 1.75
  line L210 (97.5, -897.5) -> (97.5, -882.5)
  line L211 (16.5, -573.5) -> (16.5, -558.5)
  line L212 (19.5, -963.5) -> (19.5, -1041.5) construction
  line L213 (163.5, -801.5) -> (163.5, -816.5)
  line L214 (340.5, -801.5) -> (325.5, -801.5)
  line L215 (97.5, -801.5) -> (82.5, -801.5)
  line L216 (-79.5, -558.5) -> (-79.5, -573.5)
  circle A29 centre (171, -809) radius 1.75
  line L217 (1.5, -654.5) -> (16.5, -654.5)
  line L218 (-145.5, -654.5) -> (-145.5, -639.5)
  line L219 (-142.5, -1041.5) -> (-64.5, -1041.5) construction
  line L220 (-226.5, -558.5) -> (-340.5, -558.5) construction
  line L221 (259.5, -1041.5) -> (259.5, -963.5) construction
  line L222 (-160.5, -735.5) -> (-145.5, -735.5)
  line L223 (259.5, -801.5) -> (244.5, -801.5)
  line L224 (-64.5, -801.5) -> (-79.5, -801.5)
  line L225 (1.5, -735.5) -> (16.5, -735.5)
  line L226 (-64.5, -735.5) -> (-64.5, -720.5)
  line L227 (-223.5, -558.5) -> (-226.5, -558.5)
  line L228 (-160.5, -639.5) -> (-160.5, -654.5)
  circle A30 centre (333, -890) radius 1.75
  line L229 (262.5, -1041.5) -> (340.5, -1041.5) construction
  circle A31 centre (90, -809) radius 1.75
  circle A32 centre (9, -647) radius 1.75
  circle A33 centre (333, -809) radius 1.75
  line L230 (163.5, -882.5) -> (163.5, -897.5)
  line L231 (-340.5, -717.5) -> (-340.5, -639.5)
  line L232 (340.5, -1041.5) -> (340.5, -963.5) construction
  line L233 (97.5, -816.5) -> (97.5, -801.5)
  circle A34 centre (-153, -647) radius 1.75
  line L234 (-79.5, -801.5) -> (-79.5, -816.5)
  line L235 (-145.5, -735.5) -> (-145.5, -720.5)
  line L236 (1.5, -720.5) -> (1.5, -735.5)
  line L237 (-79.5, -639.5) -> (-79.5, -654.5)
  line L238 (16.5, -801.5) -> (1.5, -801.5)
  line L239 (82.5, -801.5) -> (82.5, -816.5)
  point P0 (0, -800)
  point P1 (0, -800)
  dimension "d358" = 3.5
  dimension "d359" = 3.5
  dimension "d360" = 3.5
  dimension "d361" = 3.5
  dimension "d362" = 3.5
  dimension "d363" = 3.5
  dimension "d364" = 3.5
  dimension "d365" = 3.5
  dimension "d366" = 3.5
  dimension "d367" = 3.5
  dimension "d368" = 3.5
  dimension "d369" = 3.5
  dimension "d370" = 3.5
  dimension "d371" = 3.5
  dimension "d372" = 3.5
  dimension "d373" = 3.5
  dimension "d374" = 3.5
  dimension "d375" = 3.5
  dimension "d376" = 3.5
  dimension "d377" = 3.5
  dimension "d378" = 3.5
  dimension "d379" = 3.5
  dimension "d380" = 3.5
  dimension "d381" = 3.5
  dimension "d382" = 3.5
  dimension "d383" = 3.5
  dimension "d384" = 3.5
  dimension "d385" = 3.5
  dimension "d386" = 3.5
  dimension "d387" = 3.5
  dimension "d388" = 3.5
  dimension "d389" = 3.5
  dimension "d390" = 3.5
  dimension "d391" = 3.5
  dimension "d392" = 3.5
  measures "d358" diameter of A19
  measures "d359" diameter of A9
  measures "d360" diameter of A13
  measures "d361" diameter of A28
  measures "d362" diameter of A6
  measures "d363" diameter of A5
  measures "d364" diameter of A30
  measures "d365" diameter of A33
  measures "d366" diameter of A25
  measures "d367" diameter of A0
  measures "d368" diameter of A1
  measures "d369" diameter of A24
  measures "d370" diameter of A23
  measures "d371" diameter of A2
  measures "d372" diameter of A4
  measures "d373" diameter of A22
  measures "d374" diameter of A27
  measures "d375" diameter of A21
  measures "d376" diameter of A20
  measures "d377" diameter of A26
  measures "d378" diameter of A29
  measures "d379" diameter of A31
  measures "d380" diameter of A17
  measures "d381" diameter of A15
  measures "d382" diameter of A7
  measures "d383" diameter of A12
  measures "d384" diameter of A8
  measures "d385" diameter of A14
  measures "d386" diameter of A32
  measures "d387" diameter of A18
  measures "d388" diameter of A34
  measures "d389" diameter of A10
  measures "d390" diameter of A11
  measures "d391" diameter of A16
  measures "d392" diameter of A3
extrude "Extrude1" add sketch "Sketch1" against normal blind 3 makes body 1 at (332.9564, 0, 652.5817) makes body 2 at (332.9564, 0, 733.5817) makes body 3 at (332.9564, 0, 895.5817) makes body 4 at (9.0436, 0, 895.5817) makes body 5 at (90.0436, 0, 733.5817) makes body 6 at (9.0436, 0, 733.5817) makes body 7 at (-153.0436, 0, 560.4183) makes body 8 at (-153.0436, 0, 722.4183) makes body 9 at (-153.0436, 0, 884.4183) makes body 10 at (-71.9564, 0, 814.5817) makes body 11 at (-72.0436, 0, 652.5817) makes body 12 at (8.9564, 0, 652.5817) makes body 13 at (170.9564, 0, 722.4183) makes body 14 at (9.0436, 0, 814.5817) makes body 15 at (251.9564, 0, 895.5817) makes body 16 at (251.9564, 0, 722.4183) makes body 17 at (170.9564, 0, 560.4183) makes body 18 at (251.9564, 0, 560.4183) makes body 19 at (170.9564, 0, 652.5817) makes body 20 at (251.9564, 0, 814.5817) makes body 21 at (90.0436, 0, 895.5817) makes body 22 at (90.0436, 0, 814.5817) makes body 23 at (90.0436, 0, 571.5817) makes body 24 at (-71.9564, 0, 571.5817) makes body 25 at (-71.9564, 0, 733.5817) makes body 26 at (-153.0436, 0, 803.4183) makes body 27 at (-71.9564, 0, 895.5817) makes body 28 at (-153.0436, 0, 652.5817) makes body 29 at (9.0436, 0, 571.5817) makes body 30 at (89.9564, 0, 652.5817) makes body 31 at (170.9564, 0, 803.4183) makes body 32 at (170.9564, 0, 884.4183) makes body 33 at (332.9564, 0, 814.5817) makes body 34 at (251.9564, 0, 652.5817) makes body 35 at (332.9564, 0, 571.5817)
ref_plane "WorkPlane1" through (-153, -3, 890) normal (0, -1, 0) x (-1, 0, 0)